Autodesk Fusion 360 part; units mm, degrees
(part 3 of 8)
sketch "Sketch2 (3)" plane through (0, 0, 5) normal (0, 0, 1) x (-1, 0, 0)
  arc A0 (-62.44, 3.6948) -> (-62.5051, 2.3488) centre (0, 0) ccw
  spline S0 degree 3 poles (-62.6664, 2.1601) (-62.6409, 2.1651) (-62.6165, 2.1751) (-62.5731, 2.2037) (-62.5543, 2.2222) (-62.5291, 2.2592) (-62.5208, 2.2761) (-62.5091, 2.3116) (-62.5058, 2.3301) (-62.5051, 2.3488) knots 0 0 0 0 0.007813 0.007813 0.015626 0.015626 0.021241 0.021241 0.026855 0.026855 0.026855 0.026855
  spline S1 degree 5 poles (-62.6664, 2.1601) (-62.6671, 2.1599) (-62.685, 2.1564) (-62.72, 2.1495) (-62.7722, 2.139) (-62.8416, 2.1247) (-62.9274, 2.1065) (-63.0131, 2.0878) (-63.0988, 2.0687) (-63.1845, 2.049) (-63.2701, 2.0289) (-63.3557, 2.0082) (-63.4413, 1.9872) (-63.5268, 1.9656) (-63.6123, 1.9436) (-63.6978, 1.9212) (-63.7832, 1.8983) (-63.8686, 1.875) (-63.954, 1.8513) (-64.0393, 1.8272) (-64.1245, 1.8027) (-64.2097, 1.7777) (-64.2949, 1.7524) (-64.3801, 1.7266) (-64.4651, 1.7005) (-64.5502, 1.674) (-64.6352, 1.647) (-64.7202, 1.6198) (-64.8051, 1.5921) (-64.89, 1.5641) (-64.9748, 1.5357) (-65.0596, 1.5069) (-65.1443, 1.4778) (-65.229, 1.4483) (-65.3136, 1.4184) (-65.3982, 1.3882) (-65.4828, 1.3577) (-65.5673, 1.3268) (-65.6517, 1.2955) (-65.7361, 1.264) (-65.8205, 1.2321) (-65.9047, 1.1998) (-65.989, 1.1672) (-66.0732, 1.1343) (-66.1573, 1.1011) (-66.2414, 1.0675) (-66.3255, 1.0336) (-66.4094, 0.9994) (-66.4934, 0.9649) (-66.5772, 0.93) (-66.6611, 0.8949) (-66.7448, 0.8594) (-66.8285, 0.8236) (-66.8955, 0.7947) (-66.9456, 0.7729) (-66.9791, 0.7583) (-66.9958, 0.751) knots 0.270845 0.270845 0.270845 0.270845 0.270845 0.270845 0.271429 0.285714 0.3 0.314286 0.328571 0.342857 0.357143 0.371429 0.385714 0.4 0.414286 0.428571 0.442857 0.457143 0.471429 0.485714 0.5 0.514286 0.528571 0.542857 0.557143 0.571429 0.585714 0.6 0.614286 0.628571 0.642857 0.657143 0.671429 0.685714 0.7 0.714286 0.728571 0.742857 0.757143 0.771429 0.785714 0.8 0.814286 0.828571 0.842857 0.857143 0.871429 0.885714 0.9 0.914286 0.928571 0.942857 0.957143 0.971429 0.985714 1 1 1 1 1 1
  arc A1 (-66.9958, 0.751) -> (-66.9958, -0.751) centre (0, 0) ccw
  spline S2 degree 5 poles (-66.9958, -0.751) (-66.9791, -0.7583) (-66.9456, -0.7729) (-66.8955, -0.7947) (-66.8285, -0.8236) (-66.7448, -0.8594) (-66.6611, -0.8949) (-66.5772, -0.93) (-66.4934, -0.9649) (-66.4094, -0.9994) (-66.3255, -1.0336) (-66.2414, -1.0675) (-66.1573, -1.1011) (-66.0732, -1.1343) (-65.989, -1.1672) (-65.9047, -1.1998) (-65.8205, -1.2321) (-65.7361, -1.264) (-65.6517, -1.2955) (-65.5673, -1.3268) (-65.4828, -1.3577) (-65.3982, -1.3882) (-65.3136, -1.4184) (-65.229, -1.4483) (-65.1443, -1.4778) (-65.0596, -1.5069) (-64.9748, -1.5357) (-64.89, -1.5641) (-64.8051, -1.5921) (-64.7202, -1.6198) (-64.6352, -1.647) (-64.5502, -1.674) (-64.4651, -1.7005) (-64.3801, -1.7266) (-64.2949, -1.7524) (-64.2097, -1.7777) (-64.1245, -1.8027) (-64.0393, -1.8272) (-63.954, -1.8513) (-63.8686, -1.875) (-63.7832, -1.8983) (-63.6978, -1.9212) (-63.6123, -1.9436) (-63.5268, -1.9656) (-63.4413, -1.9872) (-63.3557, -2.0082) (-63.2701, -2.0289) (-63.1845, -2.049) (-63.0988, -2.0687) (-63.0131, -2.0878) (-62.9274, -2.1065) (-62.8416, -2.1247) (-62.7722, -2.139) (-62.72, -2.1495) (-62.685, -2.1564) (-62.6671, -2.1599) (-62.6664, -2.1601) knots -1 -1 -1 -1 -1 -1 -0.985714 -0.971429 -0.957143 -0.942857 -0.928571 -0.914286 -0.9 -0.885714 -0.871429 -0.857143 -0.842857 -0.828571 -0.814286 -0.8 -0.785714 -0.771429 -0.757143 -0.742857 -0.728571 -0.714286 -0.7 -0.685714 -0.671429 -0.657143 -0.642857 -0.628571 -0.614286 -0.6 -0.585714 -0.571429 -0.557143 -0.542857 -0.528571 -0.514286 -0.5 -0.485714 -0.471429 -0.457143 -0.442857 -0.428571 -0.414286 -0.4 -0.385714 -0.371429 -0.357143 -0.342857 -0.328571 -0.314286 -0.3 -0.285714 -0.271429 -0.270845 -0.270845 -0.270845 -0.270845 -0.270845 -0.270845
  spline S3 degree 3 poles (-62.5051, -2.3488) (-62.5061, -2.3228) (-62.5121, -2.2972) (-62.5337, -2.2498) (-62.549, -2.2284) (-62.5816, -2.1978) (-62.597, -2.1869) (-62.6303, -2.1698) (-62.6481, -2.1637) (-62.6664, -2.1601) knots 0 0 0 0 0.007813 0.007813 0.015626 0.015626 0.021241 0.021241 0.026855 0.026855 0.026855 0.026855
  arc A2 (-62.5051, -2.3488) -> (-62.44, -3.6948) centre (0, 0) ccw
  spline S4 degree 3 poles (-62.5823, -3.8982) (-62.5574, -3.8907) (-62.5341, -3.8785) (-62.4936, -3.8457) (-62.4768, -3.8255) (-62.4553, -3.7863) (-62.4486, -3.7687) (-62.4404, -3.7322) (-62.4389, -3.7134) (-62.44, -3.6948) knots 0 0 0 0 0.007813 0.007813 0.015626 0.015626 0.021241 0.021241 0.026855 0.026855 0.026855 0.026855
  spline S5 degree 5 poles (-62.5823, -3.8982) (-62.583, -3.8984) (-62.6005, -3.9036) (-62.6347, -3.9139) (-62.6856, -3.9294) (-62.7533, -3.9503) (-62.8369, -3.9767) (-62.9204, -4.0035) (-63.0039, -4.0309) (-63.0873, -4.0587) (-63.1706, -4.0871) (-63.2538, -4.1158) (-63.3369, -4.1451) (-63.42, -4.1748) (-63.503, -4.2049) (-63.5859, -4.2355) (-63.6687, -4.2665) (-63.7514, -4.2979) (-63.8341, -4.3298) (-63.9166, -4.362) (-63.9991, -4.3947) (-64.0816, -4.4277) (-64.1639, -4.4612) (-64.2461, -4.495) (-64.3283, -4.5292) (-64.4104, -4.5638) (-64.4924, -4.5988) (-64.5744, -4.6342) (-64.6562, -4.6699) (-64.738, -4.706) (-64.8197, -4.7425) (-64.9013, -4.7793) (-64.9828, -4.8165) (-65.0643, -4.854) (-65.1456, -4.8919) (-65.2269, -4.9301) (-65.3081, -4.9687) (-65.3892, -5.0076) (-65.4703, -5.0468) (-65.5512, -5.0864) (-65.6321, -5.1263) (-65.7129, -5.1665) (-65.7936, -5.2071) (-65.8742, -5.248) (-65.9547, -5.2892) (-66.0352, -5.3307) (-66.1156, -5.3725) (-66.1959, -5.4147) (-66.2761, -5.4572) (-66.3562, -5.5) (-66.4362, -5.543) (-66.5162, -5.5864) (-66.5961, -5.6301) (-66.6599, -5.6653) (-66.7077, -5.6919) (-66.7396, -5.7096) (-66.7555, -5.7185) knots 0.270845 0.270845 0.270845 0.270845 0.270845 0.270845 0.271429 0.285714 0.3 0.314286 0.328571 0.342857 0.357143 0.371429 0.385714 0.4 0.414286 0.428571 0.442857 0.457143 0.471429 0.485714 0.5 0.514286 0.528571 0.542857 0.557143 0.571429 0.585714 0.6 0.614286 0.628571 0.642857 0.657143 0.671429 0.685714 0.7 0.714286 0.728571 0.742857 0.757143 0.771429 0.785714 0.8 0.814286 0.828571 0.842857 0.857143 0.871429 0.885714 0.9 0.914286 0.928571 0.942857 0.957143 0.971429 0.985714 1 1 1 1 1 1
  arc A3 (-66.7555, -5.7185) -> (-66.6105, -7.2135) centre (0, 0) ccw
  spline S6 degree 5 poles (-66.6105, -7.2135) (-66.5932, -7.2192) (-66.5585, -7.2305) (-66.5065, -7.2474) (-66.4371, -7.2696) (-66.3503, -7.2972) (-66.2635, -7.3244) (-66.1767, -7.3513) (-66.0898, -7.3779) (-66.003, -7.4042) (-65.9161, -7.4301) (-65.8291, -7.4557) (-65.7422, -7.481) (-65.6553, -7.506) (-65.5683, -7.5306) (-65.4813, -7.5549) (-65.3943, -7.5789) (-65.3072, -7.6025) (-65.2202, -7.6258) (-65.1331, -7.6487) (-65.046, -7.6713) (-64.9589, -7.6936) (-64.8718, -7.7155) (-64.7847, -7.737) (-64.6976, -7.7582) (-64.6104, -7.779) (-64.5233, -7.7995) (-64.4361, -7.8195) (-64.3489, -7.8393) (-64.2617, -7.8586) (-64.1745, -7.8776) (-64.0873, -7.8961) (-64.0001, -7.9143) (-63.9129, -7.9321) (-63.8256, -7.9495) (-63.7384, -7.9666) (-63.6512, -7.9832) (-63.5639, -7.9994) (-63.4767, -8.0151) (-63.3895, -8.0305) (-63.3022, -8.0454) (-63.215, -8.0599) (-63.1278, -8.074) (-63.0406, -8.0877) (-62.9534, -8.1008) (-62.8662, -8.1136) (-62.779, -8.1258) (-62.6918, -8.1376) (-62.6046, -8.1489) (-62.5174, -8.1597) (-62.4303, -8.1701) (-62.3432, -8.1799) (-62.2727, -8.1874) (-62.2198, -8.1928) (-62.1842, -8.1963) (-62.1661, -8.1981) (-62.1654, -8.1982) knots -1 -1 -1 -1 -1 -1 -0.985714 -0.971429 -0.957143 -0.942857 -0.928571 -0.914286 -0.9 -0.885714 -0.871429 -0.857143 -0.842857 -0.828571 -0.814286 -0.8 -0.785714 -0.771429 -0.757143 -0.742857 -0.728571 -0.714286 -0.7 -0.685714 -0.671429 -0.657143 -0.642857 -0.628571 -0.614286 -0.6 -0.585714 -0.571429 -0.557143 -0.542857 -0.528571 -0.514286 -0.5 -0.485714 -0.471429 -0.457143 -0.442857 -0.428571 -0.414286 -0.4 -0.385714 -0.371429 -0.357143 -0.342857 -0.328571 -0.314286 -0.3 -0.285714 -0.271429 -0.270845 -0.270845 -0.270845 -0.270845 -0.270845 -0.270845
  spline S7 degree 3 poles (-61.9866, -8.3705) (-61.9901, -8.3447) (-61.9986, -8.3198) (-62.0246, -8.2747) (-62.0419, -8.2549) (-62.0773, -8.2275) (-62.0937, -8.2182) (-62.1285, -8.2044) (-62.1468, -8.2) (-62.1654, -8.1982) knots 0 0 0 0 0.007813 0.007813 0.015626 0.015626 0.021241 0.021241 0.026855 0.026855 0.026855 0.026855
  arc A4 (-61.9866, -8.3705) -> (-61.7919, -9.7038) centre (0, 0) ccw
  spline S8 degree 3 poles (-61.914, -9.9201) (-61.8898, -9.9102) (-61.8679, -9.8958) (-61.8307, -9.8593) (-61.8159, -9.8376) (-61.7983, -9.7964) (-61.7933, -9.7783) (-61.7887, -9.7411) (-61.789, -9.7223) (-61.7919, -9.7038) knots 0 0 0 0 0.007813 0.007813 0.015626 0.015626 0.021241 0.021241 0.026855 0.026855 0.026855 0.026855
  spline S9 degree 5 poles (-61.914, -9.9201) (-61.9146, -9.9203) (-61.9315, -9.9272) (-61.9645, -9.9407) (-62.0137, -9.9611) (-62.0791, -9.9884) (-62.1597, -10.0227) (-62.2403, -10.0576) (-62.3207, -10.0928) (-62.401, -10.1286) (-62.4812, -10.1648) (-62.5613, -10.2015) (-62.6412, -10.2386) (-62.721, -10.2762) (-62.8007, -10.3142) (-62.8802, -10.3526) (-62.9597, -10.3915) (-63.039, -10.4308) (-63.1182, -10.4704) (-63.1973, -10.5105) (-63.2762, -10.551) (-63.3551, -10.5918) (-63.4338, -10.633) (-63.5124, -10.6747) (-63.5909, -10.7167) (-63.6693, -10.759) (-63.7475, -10.8018) (-63.8256, -10.8449) (-63.9037, -10.8884) (-63.9816, -10.9322) (-64.0594, -10.9763) (-64.137, -11.0209) (-64.2146, -11.0657) (-64.292, -11.111) (-64.3694, -11.1565) (-64.4466, -11.2024) (-64.5237, -11.2486) (-64.6007, -11.2952) (-64.6775, -11.342) (-64.7543, -11.3892) (-64.8309, -11.4368) (-64.9075, -11.4846) (-64.9839, -11.5328) (-65.0602, -11.5813) (-65.1364, -11.63) (-65.2124, -11.6791) (-65.2884, -11.7285) (-65.3642, -11.7783) (-65.44, -11.8283) (-65.5156, -11.8786) (-65.5911, -11.9292) (-65.6665, -11.9801) (-65.7418, -12.0313) (-65.8019, -12.0725) (-65.847, -12.1035) (-65.877, -12.1243) (-65.892, -12.1347) knots 0.270845 0.270845 0.270845 0.270845 0.270845 0.270845 0.271429 0.285714 0.3 0.314286 0.328571 0.342857 0.357143 0.371429 0.385714 0.4 0.414286 0.428571 0.442857 0.457143 0.471429 0.485714 0.5 0.514286 0.528571 0.542857 0.557143 0.571429 0.585714 0.6 0.614286 0.628571 0.642857 0.657143 0.671429 0.685714 0.7 0.714286 0.728571 0.742857 0.757143 0.771429 0.785714 0.8 0.814286 0.828571 0.842857 0.857143 0.871429 0.885714 0.9 0.914286 0.928571 0.942857 0.957143 0.971429 0.985714 1 1 1 1 1 1
  arc A5 (-65.892, -12.1347) -> (-65.6034, -13.6087) centre (0, 0) ccw
  spline S10 degree 5 poles (-65.6034, -13.6087) (-65.5856, -13.6127) (-65.55, -13.6206) (-65.4965, -13.6323) (-65.4253, -13.6478) (-65.3363, -13.6668) (-65.2473, -13.6856) (-65.1582, -13.704) (-65.0692, -13.722) (-64.9802, -13.7398) (-64.8912, -13.7572) (-64.8023, -13.7744) (-64.7133, -13.7911) (-64.6243, -13.8076) (-64.5354, -13.8237) (-64.4464, -13.8395) (-64.3575, -13.855) (-64.2686, -13.8701) (-64.1797, -13.8849) (-64.0908, -13.8993) (-64.002, -13.9134) (-63.9132, -13.9271) (-63.8243, -13.9405) (-63.7355, -13.9535) (-63.6468, -13.9662) (-63.558, -13.9785) (-63.4693, -13.9904) (-63.3806, -14.002) (-63.2919, -14.0132) (-63.2032, -14.0241) (-63.1146, -14.0345) (-63.026, -14.0446) (-62.9375, -14.0543) (-62.8489, -14.0636) (-62.7604, -14.0725) (-62.672, -14.081) (-62.5835, -14.0891) (-62.4952, -14.0968) (-62.4068, -14.1041) (-62.3185, -14.111) (-62.2302, -14.1174) (-62.142, -14.1235) (-62.0538, -14.129) (-61.9657, -14.1342) (-61.8776, -14.1389) (-61.7896, -14.1432) (-61.7016, -14.1469) (-61.6137, -14.1503) (-61.5258, -14.1531) (-61.438, -14.1554) (-61.3503, -14.1573) (-61.2626, -14.1587) (-61.1918, -14.1594) (-61.1386, -14.1596) (-61.1029, -14.1597) (-61.0847, -14.1597) (-61.0839, -14.1597) knots -1 -1 -1 -1 -1 -1 -0.985714 -0.971429 -0.957143 -0.942857 -0.928571 -0.914286 -0.9 -0.885714 -0.871429 -0.857143 -0.842857 -0.828571 -0.814286 -0.8 -0.785714 -0.771429 -0.757143 -0.742857 -0.728571 -0.714286 -0.7 -0.685714 -0.671429 -0.657143 -0.642857 -0.628571 -0.614286 -0.6 -0.585714 -0.571429 -0.557143 -0.542857 -0.528571 -0.514286 -0.5 -0.485714 -0.471429 -0.457143 -0.442857 -0.428571 -0.414286 -0.4 -0.385714 -0.371429 -0.357143 -0.342857 -0.328571 -0.314286 -0.3 -0.285714 -0.271429 -0.270845 -0.270845 -0.270845 -0.270845 -0.270845 -0.270845
  spline S11 degree 3 poles (-60.8894, -14.314) (-60.8953, -14.2886) (-60.9062, -14.2647) (-60.9364, -14.2223) (-60.9556, -14.2042) (-60.9935, -14.1804) (-61.0106, -14.1727) (-61.0466, -14.1624) (-61.0652, -14.1597) (-61.0839, -14.1597) knots 0 0 0 0 0.007813 0.007813 0.015626 0.015626 0.021241 0.021241 0.026855 0.026855 0.026855 0.026855
  arc A6 (-60.8894, -14.314) -> (-60.5669, -15.6223) centre (0, 0) ccw
  spline S12 degree 3 poles (-60.6675, -15.8493) (-60.6444, -15.8372) (-60.624, -15.8207) (-60.5905, -15.7808) (-60.5778, -15.7577) (-60.5643, -15.7151) (-60.5611, -15.6965) (-60.5601, -15.6591) (-60.5622, -15.6404) (-60.5669, -15.6223) knots 0 0 0 0 0.007813 0.007813 0.015626 0.015626 0.021241 0.021241 0.026855 0.026855 0.026855 0.026855
  spline S13 degree 5 poles (-60.6675, -15.8493) (-60.6681, -15.8496) (-60.6843, -15.8581) (-60.7158, -15.8748) (-60.7629, -15.8998) (-60.8252, -15.9333) (-60.9022, -15.9752) (-60.9791, -16.0177) (-61.0557, -16.0605) (-61.1322, -16.1039) (-61.2085, -16.1477) (-61.2846, -16.1919) (-61.3606, -16.2366) (-61.4364, -16.2817) (-61.512, -16.3272) (-61.5875, -16.3731) (-61.6628, -16.4195) (-61.738, -16.4662) (-61.813, -16.5133) (-61.8878, -16.5608) (-61.9625, -16.6087) (-62.037, -16.657) (-62.1114, -16.7057) (-62.1856, -16.7547) (-62.2597, -16.804) (-62.3336, -16.8538) (-62.4074, -16.9039) (-62.481, -16.9543) (-62.5545, -17.0051) (-62.6278, -17.0563) (-62.7009, -17.1077) (-62.7739, -17.1595) (-62.8468, -17.2117) (-62.9195, -17.2642) (-62.9921, -17.317) (-63.0645, -17.3701) (-63.1368, -17.4235) (-63.2089, -17.4773) (-63.2809, -17.5314) (-63.3528, -17.5858) (-63.4245, -17.6405) (-63.496, -17.6955) (-63.5674, -17.7508) (-63.6387, -17.8064) (-63.7098, -17.8623) (-63.7808, -17.9185) (-63.8516, -17.975) (-63.9223, -18.0318) (-63.9929, -18.0889) (-64.0633, -18.1463) (-64.1336, -18.204) (-64.2037, -18.2619) (-64.2737, -18.3201) (-64.3296, -18.3669) (-64.3714, -18.4022) (-64.3993, -18.4257) (-64.4132, -18.4375) knots 0.270845 0.270845 0.270845 0.270845 0.270845 0.270845 0.271429 0.285714 0.3 0.314286 0.328571 0.342857 0.357143 0.371429 0.385714 0.4 0.414286 0.428571 0.442857 0.457143 0.471429 0.485714 0.5 0.514286 0.528571 0.542857 0.557143 0.571429 0.585714 0.6 0.614286 0.628571 0.642857 0.657143 0.671429 0.685714 0.7 0.714286 0.728571 0.742857 0.757143 0.771429 0.785714 0.8 0.814286 0.828571 0.842857 0.857143 0.871429 0.885714 0.9 0.914286 0.928571 0.942857 0.957143 0.971429 0.985714 1 1 1 1 1 1
  arc A7 (-64.4132, -18.4375) -> (-63.9837, -19.8768) centre (0, 0) ccw
  spline S14 degree 5 poles (-63.9837, -19.8768) (-63.9656, -19.879) (-63.9294, -19.8835) (-63.8751, -19.89) (-63.8027, -19.8985) (-63.7122, -19.9089) (-63.6218, -19.9189) (-63.5314, -19.9287) (-63.4411, -19.9381) (-63.3508, -19.9472) (-63.2605, -19.9559) (-63.1703, -19.9644) (-63.0801, -19.9725) (-62.99, -19.9803) (-62.8999, -19.9877) (-62.8099, -19.9949) (-62.7199, -20.0017) (-62.6299, -20.0081) (-62.54, -20.0143) (-62.4502, -20.0201) (-62.3604, -20.0255) (-62.2706, -20.0306) (-62.1809, -20.0353) (-62.0913, -20.0397) (-62.0017, -20.0438) (-61.9122, -20.0475) (-61.8227, -20.0508) (-61.7333, -20.0538) (-61.644, -20.0564) (-61.5547, -20.0586) (-61.4655, -20.0604) (-61.3763, -20.0619) (-61.2872, -20.063) (-61.1982, -20.0637) (-61.1093, -20.0641) (-61.0204, -20.064) (-60.9316, -20.0635) (-60.8429, -20.0627) (-60.7542, -20.0614) (-60.6657, -20.0597) (-60.5772, -20.0576) (-60.4888, -20.0551) (-60.4005, -20.0521) (-60.3123, -20.0488) (-60.2242, -20.045) (-60.1361, -20.0407) (-60.0482, -20.036) (-59.9604, -20.0308) (-59.8726, -20.0251) (-59.785, -20.019) (-59.6975, -20.0124) (-59.6101, -20.0053) (-59.5396, -19.9991) (-59.4866, -19.9943) (-59.451, -19.9909) (-59.4329, -19.9891) (-59.4322, -19.9891) knots -1 -1 -1 -1 -1 -1 -0.985714 -0.971429 -0.957143 -0.942857 -0.928571 -0.914286 -0.9 -0.885714 -0.871429 -0.857143 -0.842857 -0.828571 -0.814286 -0.8 -0.785714 -0.771429 -0.757143 -0.742857 -0.728571 -0.714286 -0.7 -0.685714 -0.671429 -0.657143 -0.642857 -0.628571 -0.614286 -0.6 -0.585714 -0.571429 -0.557143 -0.542857 -0.528571 -0.514286 -0.5 -0.485714 -0.471429 -0.457143 -0.442857 -0.428571 -0.414286 -0.4 -0.385714 -0.371429 -0.357143 -0.342857 -0.328571 -0.314286 -0.3 -0.285714 -0.271429 -0.270845 -0.270845 -0.270845 -0.270845 -0.270845 -0.270845
  spline S15 degree 3 poles (-59.2236, -20.1238) (-59.232, -20.0991) (-59.2451, -20.0764) (-59.2793, -20.0371) (-59.3001, -20.021) (-59.3401, -20.001) (-59.3579, -19.995) (-59.3947, -19.9881) (-59.4135, -19.9873) (-59.4322, -19.9891) knots 0 0 0 0 0.007813 0.007813 0.015626 0.015626 0.021241 0.021241 0.026855 0.026855 0.026855 0.026855
  arc A8 (-59.2236, -20.1238) -> (-58.7764, -21.3949) centre (0, 0) ccw
  spline S16 degree 3 poles (-58.8546, -21.6306) (-58.8328, -21.6163) (-58.814, -21.5979) (-58.7846, -21.5549) (-58.7742, -21.5308) (-58.7648, -21.487) (-58.7635, -21.4683) (-58.766, -21.4309) (-58.77, -21.4125) (-58.7764, -21.3949) knots 0 0 0 0 0.007813 0.007813 0.015626 0.015626 0.021241 0.021241 0.026855 0.026855 0.026855 0.026855
  spline S17 degree 5 poles (-58.8546, -21.6306) (-58.8552, -21.631) (-58.8704, -21.641) (-58.9003, -21.6606) (-58.9447, -21.69) (-59.0035, -21.7294) (-59.0761, -21.7786) (-59.1485, -21.8282) (-59.2206, -21.8783) (-59.2925, -21.9288) (-59.3643, -21.9798) (-59.4358, -22.0311) (-59.5071, -22.0829) (-59.5782, -22.1351) (-59.6491, -22.1878) (-59.7198, -22.2408) (-59.7903, -22.2941) (-59.8606, -22.3479) (-59.9307, -22.402) (-60.0006, -22.4566) (-60.0703, -22.5114) (-60.1398, -22.5667) (-60.2091, -22.6223) (-60.2783, -22.6782) (-60.3472, -22.7345) (-60.416, -22.7912) (-60.4846, -22.8481) (-60.553, -22.9055) (-60.6212, -22.9631) (-60.6892, -23.0211) (-60.7571, -23.0794) (-60.8248, -23.138) (-60.8923, -23.1969) (-60.9596, -23.2562) (-61.0267, -23.3157) (-61.0937, -23.3756) (-61.1605, -23.4358) (-61.2271, -23.4962) (-61.2935, -23.557) (-61.3597, -23.6181) (-61.4258, -23.6795) (-61.4917, -23.7411) (-61.5575, -23.8031) (-61.623, -23.8653) (-61.6884, -23.9278) (-61.7537, -23.9906) (-61.8187, -24.0537) (-61.8836, -24.117) (-61.9483, -24.1807) (-62.0129, -24.2446) (-62.0772, -24.3088) (-62.1414, -24.3732) (-62.2055, -24.4379) (-62.2566, -24.4899) (-62.2948, -24.529) (-62.3203, -24.5551) (-62.333, -24.5682) knots 0.270845 0.270845 0.270845 0.270845 0.270845 0.270845 0.271429 0.285714 0.3 0.314286 0.328571 0.342857 0.357143 0.371429 0.385714 0.4 0.414286 0.428571 0.442857 0.457143 0.471429 0.485714 0.5 0.514286 0.528571 0.542857 0.557143 0.571429 0.585714 0.6 0.614286 0.628571 0.642857 0.657143 0.671429 0.685714 0.7 0.714286 0.728571 0.742857 0.757143 0.771429 0.785714 0.8 0.814286 0.828571 0.842857 0.857143 0.871429 0.885714 0.9 0.914286 0.928571 0.942857 0.957143 0.971429 0.985714 1 1 1 1 1 1
  arc A9 (-62.333, -24.5682) -> (-61.7666, -25.9593) centre (0, 0) ccw
  spline S18 degree 5 poles (-61.7666, -25.9593) (-61.7484, -25.9598) (-61.7119, -25.9607) (-61.6572, -25.962) (-61.5843, -25.9635) (-61.4933, -25.9651) (-61.4023, -25.9663) (-61.3114, -25.9673) (-61.2206, -25.9679) (-61.1299, -25.9683) (-61.0392, -25.9683) (-60.9486, -25.968) (-60.858, -25.9674) (-60.7676, -25.9664) (-60.6772, -25.9652) (-60.5869, -25.9636) (-60.4966, -25.9616) (-60.4065, -25.9594) (-60.3164, -25.9568) (-60.2264, -25.9539) (-60.1365, -25.9507) (-60.0467, -25.9471) (-59.957, -25.9431) (-59.8673, -25.9389) (-59.7778, -25.9342) (-59.6883, -25.9293) (-59.5989, -25.9239) (-59.5096, -25.9183) (-59.4205, -25.9122) (-59.3314, -25.9058) (-59.2424, -25.8991) (-59.1535, -25.8919) (-59.0647, -25.8844) (-58.9761, -25.8765) (-58.8875, -25.8683) (-58.7991, -25.8596) (-58.7107, -25.8506) (-58.6225, -25.8412) (-58.5344, -25.8314) (-58.4464, -25.8211) (-58.3586, -25.8105) (-58.2708, -25.7995) (-58.1832, -25.788) (-58.0957, -25.7761) (-58.0084, -25.7638) (-57.9212, -25.7511) (-57.8341, -25.7379) (-57.7472, -25.7243) (-57.6604, -25.7102) (-57.5738, -25.6956) (-57.4874, -25.6806) (-57.4011, -25.6651) (-57.3315, -25.6522) (-57.2791, -25.6422) (-57.2441, -25.6354) (-57.2262, -25.6319) (-57.2255, -25.6318) knots -1 -1 -1 -1 -1 -1 -0.985714 -0.971429 -0.957143 -0.942857 -0.928571 -0.914286 -0.9 -0.885714 -0.871429 -0.857143 -0.842857 -0.828571 -0.814286 -0.8 -0.785714 -0.771429 -0.757143 -0.742857 -0.728571 -0.714286 -0.7 -0.685714 -0.671429 -0.657143 -0.642857 -0.628571 -0.614286 -0.6 -0.585714 -0.571429 -0.557143 -0.542857 -0.528571 -0.514286 -0.5 -0.485714 -0.471429 -0.457143 -0.442857 -0.428571 -0.414286 -0.4 -0.385714 -0.371429 -0.357143 -0.342857 -0.328571 -0.314286 -0.3 -0.285714 -0.271429 -0.270845 -0.270845 -0.270845 -0.270845 -0.270845 -0.270845
  spline S19 degree 3 poles (-57.0049, -25.7458) (-57.0156, -25.722) (-57.0309, -25.7006) (-57.0687, -25.6648) (-57.091, -25.6508) (-57.1327, -25.6347) (-57.1511, -25.6305) (-57.1883, -25.6272) (-57.2071, -25.6282) (-57.2255, -25.6318) knots 0 0 0 0 0.007813 0.007813 0.015626 0.015626 0.021241 0.021241 0.026855 0.026855 0.026855 0.026855
  arc A10 (-57.0049, -25.7458) -> (-56.4371, -26.9678) centre (0, 0) ccw
  spline S20 degree 3 poles (-56.4922, -27.2099) (-56.4719, -27.1936) (-56.455, -27.1734) (-56.4298, -27.1278) (-56.4218, -27.1028) (-56.4167, -27.0583) (-56.4172, -27.0395) (-56.4233, -27.0026) (-56.429, -26.9847) (-56.4371, -26.9678) knots 0 0 0 0 0.007813 0.007813 0.015626 0.015626 0.021241 0.021241 0.026855 0.026855 0.026855 0.026855
  spline S21 degree 5 poles (-56.4922, -27.2099) (-56.4928, -27.2103) (-56.5069, -27.2217) (-56.5347, -27.2442) (-56.5761, -27.2777) (-56.6309, -27.3226) (-56.6984, -27.3786) (-56.7656, -27.435) (-56.8326, -27.4918) (-56.8993, -27.549) (-56.9658, -27.6066) (-57.032, -27.6647) (-57.098, -27.7231) (-57.1637, -27.7819) (-57.2292, -27.8411) (-57.2944, -27.9007) (-57.3594, -27.9607) (-57.4242, -28.021) (-57.4888, -28.0816) (-57.5531, -28.1426) (-57.6172, -28.204) (-57.681, -28.2657) (-57.7447, -28.3277) (-57.8081, -28.3901) (-57.8713, -28.4527) (-57.9343, -28.5158) (-57.9971, -28.5791) (-58.0596, -28.6427) (-58.1219, -28.7067) (-58.1841, -28.771) (-58.246, -28.8355) (-58.3077, -28.9004) (-58.3692, -28.9656) (-58.4304, -29.0311) (-58.4915, -29.0968) (-58.5524, -29.1629) (-58.6131, -29.2292) (-58.6735, -29.2958) (-58.7338, -29.3627) (-58.7938, -29.4299) (-58.8537, -29.4974) (-58.9133, -29.5651) (-58.9728, -29.6331) (-59.032, -29.7014) (-59.0911, -29.7699) (-59.15, -29.8387) (-59.2086, -29.9078) (-59.2671, -29.9771) (-59.3253, -30.0467) (-59.3834, -30.1165) (-59.4413, -30.1866) (-59.499, -30.2569) (-59.5565, -30.3275) (-59.6023, -30.3842) (-59.6366, -30.4268) (-59.6594, -30.4553) (-59.6708, -30.4695) knots 0.270845 0.270845 0.270845 0.270845 0.270845 0.270845 0.271429 0.285714 0.3 0.314286 0.328571 0.342857 0.357143 0.371429 0.385714 0.4 0.414286 0.428571 0.442857 0.457143 0.471429 0.485714 0.5 0.514286 0.528571 0.542857 0.557143 0.571429 0.585714 0.6 0.614286 0.628571 0.642857 0.657143 0.671429 0.685714 0.7 0.714286 0.728571 0.742857 0.757143 0.771429 0.785714 0.8 0.814286 0.828571 0.842857 0.857143 0.871429 0.885714 0.9 0.914286 0.928571 0.942857 0.957143 0.971429 0.985714 1 1 1 1 1 1
  arc A11 (-59.6708, -30.4695) -> (-58.9728, -31.7995) centre (0, 0) ccw
  spline S22 degree 5 poles (-58.9728, -31.7995) (-58.9546, -31.7982) (-58.9182, -31.7956) (-58.8637, -31.7916) (-58.791, -31.786) (-58.7002, -31.7788) (-58.6096, -31.7713) (-58.519, -31.7635) (-58.4286, -31.7554) (-58.3382, -31.7469) (-58.2479, -31.7382) (-58.1578, -31.7291) (-58.0677, -31.7198) (-57.9778, -31.7101) (-57.8879, -31.7001) (-57.7982, -31.6898) (-57.7086, -31.6792) (-57.619, -31.6683) (-57.5296, -31.657) (-57.4403, -31.6454) (-57.3512, -31.6335) (-57.2621, -31.6213) (-57.1732, -31.6087) (-57.0844, -31.5958) (-56.9957, -31.5826) (-56.9071, -31.569) (-56.8187, -31.555) (-56.7304, -31.5408) (-56.6422, -31.5262) (-56.5541, -31.5112) (-56.4662, -31.4959) (-56.3784, -31.4802) (-56.2908, -31.4642) (-56.2033, -31.4478) (-56.116, -31.431) (-56.0288, -31.4138) (-55.9417, -31.3963) (-55.8548, -31.3784) (-55.7681, -31.3602) (-55.6815, -31.3415) (-55.595, -31.3224) (-55.5088, -31.303) (-55.4227, -31.2831) (-55.3368, -31.2629) (-55.251, -31.2422) (-55.1654, -31.2211) (-55.0801, -31.1996) (-54.9949, -31.1776) (-54.9099, -31.1552) (-54.8251, -31.1323) (-54.7405, -31.109) (-54.6561, -31.0853) (-54.588, -31.0657) (-54.5369, -31.0507) (-54.5027, -31.0406) (-54.4852, -31.0354) (-54.4845, -31.0352) knots -1 -1 -1 -1 -1 -1 -0.985714 -0.971429 -0.957143 -0.942857 -0.928571 -0.914286 -0.9 -0.885714 -0.871429 -0.857143 -0.842857 -0.828571 -0.814286 -0.8 -0.785714 -0.771429 -0.757143 -0.742857 -0.728571 -0.714286 -0.7 -0.685714 -0.671429 -0.657143 -0.642857 -0.628571 -0.614286 -0.6 -0.585714 -0.571429 -0.557143 -0.542857 -0.528571 -0.514286 -0.5 -0.485714 -0.471429 -0.457143 -0.442857 -0.428571 -0.414286 -0.4 -0.385714 -0.371429 -0.357143 -0.342857 -0.328571 -0.314286 -0.3 -0.285714 -0.271429 -0.270845 -0.270845 -0.270845 -0.270845 -0.270845 -0.270845
  spline S23 degree 3 poles (-54.254, -31.1273) (-54.2669, -31.1047) (-54.2842, -31.0849) (-54.3253, -31.053) (-54.3488, -31.0411) (-54.3919, -31.0292) (-54.4106, -31.0267) (-54.448, -31.027) (-54.4666, -31.0298) (-54.4845, -31.0352) knots 0 0 0 0 0.007813 0.007813 0.015626 0.015626 0.021241 0.021241 0.026855 0.026855 0.026855 0.026855
  arc A12 (-54.254, -31.1273) -> (-53.5708, -32.2888) centre (0, 0) ccw
  spline S24 degree 3 poles (-53.6023, -32.5351) (-53.5837, -32.5169) (-53.5688, -32.4953) (-53.5482, -32.4475) (-53.5426, -32.4218) (-53.5418, -32.377) (-53.5441, -32.3583) (-53.5538, -32.3222) (-53.5612, -32.3049) (-53.5708, -32.2888) knots 0 0 0 0 0.007813 0.007813 0.015626 0.015626 0.021241 0.021241 0.026855 0.026855 0.026855 0.026855
  spline S25 degree 5 poles (-53.6023, -32.5351) (-53.6028, -32.5356) (-53.6159, -32.5484) (-53.6414, -32.5734) (-53.6793, -32.6108) (-53.7295, -32.6607) (-53.7913, -32.7229) (-53.8527, -32.7856) (-53.9139, -32.8486) (-53.9748, -32.912) (-54.0354, -32.9757) (-54.0957, -33.0399) (-54.1558, -33.1044) (-54.2155, -33.1693) (-54.275, -33.2346) (-54.3342, -33.3002) (-54.3931, -33.3661) (-54.4517, -33.4324) (-54.5101, -33.499) (-54.5683, -33.5659) (-54.6261, -33.6332) (-54.6837, -33.7007) (-54.7411, -33.7686) (-54.7982, -33.8368) (-54.8551, -33.9053) (-54.9117, -33.9741) (-54.968, -34.0432) (-55.0241, -34.1126) (-55.08, -34.1823) (-55.1356, -34.2522) (-55.191, -34.3225) (-55.2462, -34.393) (-55.3011, -34.4638) (-55.3558, -34.5349) (-55.4102, -34.6062) (-55.4644, -34.6778) (-55.5184, -34.7497) (-55.5721, -34.8219) (-55.6257, -34.8943) (-55.679, -34.9669) (-55.732, -35.0399) (-55.7849, -35.113) (-55.8375, -35.1864) (-55.8899, -35.2601) (-55.942, -35.334) (-55.994, -35.4082) (-56.0457, -35.4826) (-56.0972, -35.5572) (-56.1485, -35.6321) (-56.1995, -35.7072) (-56.2504, -35.7826) (-56.301, -35.8582) (-56.3514, -35.934) (-56.3916, -35.9948) (-56.4216, -36.0405) (-56.4416, -36.0711) (-56.4515, -36.0863) knots 0.270845 0.270845 0.270845 0.270845 0.270845 0.270845 0.271429 0.285714 0.3 0.314286 0.328571 0.342857 0.357143 0.371429 0.385714 0.4 0.414286 0.428571 0.442857 0.457143 0.471429 0.485714 0.5 0.514286 0.528571 0.542857 0.557143 0.571429 0.585714 0.6 0.614286 0.628571 0.642857 0.657143 0.671429 0.685714 0.7 0.714286 0.728571 0.742857 0.757143 0.771429 0.785714 0.8 0.814286 0.828571 0.842857 0.857143 0.871429 0.885714 0.9 0.914286 0.928571 0.942857 0.957143 0.971429 0.985714 1 1 1 1 1 1
  arc A13 (-56.4515, -36.0863) -> (-55.6284, -37.3427) centre (0, 0) ccw
  spline S26 degree 5 poles (-55.6284, -37.3427) (-55.6104, -37.3397) (-55.5745, -37.3336) (-55.5205, -37.3243) (-55.4487, -37.3118) (-55.3591, -37.2958) (-55.2696, -37.2796) (-55.1802, -37.2631) (-55.091, -37.2463) (-55.0018, -37.2292) (-54.9128, -37.2118) (-54.824, -37.1941) (-54.7352, -37.176) (-54.6466, -37.1577) (-54.5582, -37.1391) (-54.4698, -37.1202) (-54.3817, -37.101) (-54.2936, -37.0815) (-54.2057, -37.0616) (-54.118, -37.0415) (-54.0304, -37.021) (-53.9429, -37.0002) (-53.8556, -36.9791) (-53.7684, -36.9577) (-53.6814, -36.936) (-53.5946, -36.9139) (-53.5079, -36.8915) (-53.4214, -36.8688) (-53.335, -36.8457) (-53.2488, -36.8223) (-53.1628, -36.7986) (-53.077, -36.7745) (-52.9913, -36.7501) (-52.9058, -36.7253) (-52.8205, -36.7002) (-52.7353, -36.6747) (-52.6504, -36.6489) (-52.5656, -36.6227) (-52.481, -36.5962) (-52.3966, -36.5692) (-52.3125, -36.5419) (-52.2285, -36.5142) (-52.1447, -36.4861) (-52.0611, -36.4577) (-51.9778, -36.4288) (-51.8946, -36.3996) (-51.8117, -36.3699) (-51.7291, -36.3398) (-51.6466, -36.3093) (-51.5644, -36.2784) (-51.4825, -36.247) (-51.4007, -36.2152) (-51.3349, -36.1892) (-51.2855, -36.1693) (-51.2524, -36.1559) (-51.2355, -36.1491) (-51.2348, -36.1488) knots -1 -1 -1 -1 -1 -1 -0.985714 -0.971429 -0.957143 -0.942857 -0.928571 -0.914286 -0.9 -0.885714 -0.871429 -0.857143 -0.842857 -0.828571 -0.814286 -0.8 -0.785714 -0.771429 -0.757143 -0.742857 -0.728571 -0.714286 -0.7 -0.685714 -0.671429 -0.657143 -0.642857 -0.628571 -0.614286 -0.6 -0.585714 -0.571429 -0.557143 -0.542857 -0.528571 -0.514286 -0.5 -0.485714 -0.471429 -0.457143 -0.442857 -0.428571 -0.414286 -0.4 -0.385714 -0.371429 -0.357143 -0.342857 -0.328571 -0.314286 -0.3 -0.285714 -0.271429 -0.270845 -0.270845 -0.270845 -0.270845 -0.270845 -0.270845
  spline S27 degree 3 poles (-50.9965, -36.2183) (-51.0115, -36.1971) (-51.0306, -36.179) (-51.0746, -36.1511) (-51.0992, -36.1416) (-51.1432, -36.1339) (-51.162, -36.1332) (-51.1993, -36.1372) (-51.2175, -36.1418) (-51.2348, -36.1488) knots 0 0 0 0 0.007813 0.007813 0.015626 0.015626 0.021241 0.021241 0.026855 0.026855 0.026855 0.026855
  arc A14 (-50.9965, -36.2183) -> (-50.2044, -37.3084) centre (0, 0) ccw
  spline S28 degree 3 poles (-50.212, -37.5566) (-50.1952, -37.5367) (-50.1825, -37.5137) (-50.1666, -37.4641) (-50.1635, -37.438) (-50.167, -37.3934) (-50.1711, -37.375) (-50.1842, -37.34) (-50.1932, -37.3235) (-50.2044, -37.3084) knots 0 0 0 0 0.007813 0.007813 0.015626 0.015626 0.021241 0.021241 0.026855 0.026855 0.026855 0.026855
  spline S29 degree 5 poles (-50.212, -37.5566) (-50.2125, -37.5572) (-50.2242, -37.5711) (-50.2472, -37.5985) (-50.2813, -37.6393) (-50.3264, -37.6939) (-50.3819, -37.7618) (-50.4371, -37.83) (-50.4919, -37.8987) (-50.5464, -37.9676) (-50.6005, -38.037) (-50.6544, -38.1067) (-50.7079, -38.1767) (-50.7611, -38.247) (-50.814, -38.3177) (-50.8666, -38.3887) (-50.9189, -38.46) (-50.9708, -38.5317) (-51.0225, -38.6036) (-51.0739, -38.6758) (-51.125, -38.7483) (-51.1759, -38.8211) (-51.2264, -38.8942) (-51.2767, -38.9676) (-51.3266, -39.0413) (-51.3763, -39.1152) (-51.4258, -39.1894) (-51.4749, -39.2639) (-51.5238, -39.3387) (-51.5724, -39.4137) (-51.6208, -39.4889) (-51.6689, -39.5645) (-51.7167, -39.6402) (-51.7643, -39.7163) (-51.8116, -39.7925) (-51.8586, -39.869) (-51.9054, -39.9458) (-51.9519, -40.0228) (-51.9982, -40.1) (-52.0442, -40.1775) (-52.09, -40.2552) (-52.1355, -40.3331) (-52.1808, -40.4113) (-52.2259, -40.4897) (-52.2706, -40.5683) (-52.3152, -40.6471) (-52.3595, -40.7261) (-52.4035, -40.8054) (-52.4474, -40.8849) (-52.4909, -40.9646) (-52.5343, -41.0445) (-52.5774, -41.1246) (-52.6202, -41.2049) (-52.6543, -41.2693) (-52.6798, -41.3177) (-52.6967, -41.3501) (-52.7052, -41.3662) knots 0.270845 0.270845 0.270845 0.270845 0.270845 0.270845 0.271429 0.285714 0.3 0.314286 0.328571 0.342857 0.357143 0.371429 0.385714 0.4 0.414286 0.428571 0.442857 0.457143 0.471429 0.485714 0.5 0.514286 0.528571 0.542857 0.557143 0.571429 0.585714 0.6 0.614286 0.628571 0.642857 0.657143 0.671429 0.685714 0.7 0.714286 0.728571 0.742857 0.757143 0.771429 0.785714 0.8 0.814286 0.828571 0.842857 0.857143 0.871429 0.885714 0.9 0.914286 0.928571 0.942857 0.957143 0.971429 0.985714 1 1 1 1 1 1
  arc A15 (-52.7052, -41.3662) -> (-51.7646, -42.5373) centre (0, 0) ccw
  spline S30 degree 5 poles (-51.7646, -42.5373) (-51.747, -42.5326) (-51.7118, -42.523) (-51.659, -42.5086) (-51.5888, -42.4892) (-51.5011, -42.4647) (-51.4136, -42.4399) (-51.3262, -42.4148) (-51.239, -42.3894) (-51.1519, -42.3638) (-51.065, -42.3379) (-50.9783, -42.3117) (-50.8917, -42.2852) (-50.8053, -42.2584) (-50.719, -42.2314) (-50.6329, -42.204) (-50.547, -42.1764) (-50.4613, -42.1485) (-50.3757, -42.1202) (-50.2903, -42.0917) (-50.2051, -42.0629) (-50.12, -42.0338) (-50.0352, -42.0043) (-49.9505, -41.9746) (-49.866, -41.9446) (-49.7817, -41.9142) (-49.6976, -41.8836) (-49.6136, -41.8526) (-49.5299, -41.8213) (-49.4464, -41.7897) (-49.3631, -41.7578) (-49.2799, -41.7255) (-49.197, -41.6929) (-49.1143, -41.66) (-49.0318, -41.6268) (-48.9495, -41.5932) (-48.8674, -41.5593) (-48.7856, -41.5251) (-48.704, -41.4905) (-48.6226, -41.4555) (-48.5414, -41.4202) (-48.4605, -41.3845) (-48.3798, -41.3485) (-48.2994, -41.3121) (-48.2192, -41.2753) (-48.1393, -41.2382) (-48.0597, -41.2007) (-47.9803, -41.1628) (-47.9012, -41.1244) (-47.8223, -41.0857) (-47.7438, -41.0466) (-47.6655, -41.007) (-47.6025, -40.9748) (-47.5552, -40.9503) (-47.5236, -40.9337) (-47.5074, -40.9253) (-47.5068, -40.9249) knots -1 -1 -1 -1 -1 -1 -0.985714 -0.971429 -0.957143 -0.942857 -0.928571 -0.914286 -0.9 -0.885714 -0.871429 -0.857143 -0.842857 -0.828571 -0.814286 -0.8 -0.785714 -0.771429 -0.757143 -0.742857 -0.728571 -0.714286 -0.7 -0.685714 -0.671429 -0.657143 -0.642857 -0.628571 -0.614286 -0.6 -0.585714 -0.571429 -0.557143 -0.542857 -0.528571 -0.514286 -0.5 -0.485714 -0.471429 -0.457143 -0.442857 -0.428571 -0.414286 -0.4 -0.385714 -0.371429 -0.357143 -0.342857 -0.328571 -0.314286 -0.3 -0.285714 -0.271429 -0.270845 -0.270845 -0.270845 -0.270845 -0.270845 -0.270845
  spline S31 degree 3 poles (-47.2628, -40.9711) (-47.2799, -40.9514) (-47.3006, -40.9352) (-47.3471, -40.9118) (-47.3724, -40.9047) (-47.4171, -40.9012) (-47.4358, -40.9024) (-47.4725, -40.9099) (-47.4902, -40.9163) (-47.5068, -40.9249) knots 0 0 0 0 0.007813 0.007813 0.015626 0.015626 0.021241 0.021241 0.026855 0.026855 0.026855 0.026855
  arc A16 (-47.2628, -40.9711) -> (-46.3693, -41.9797) centre (0, 0) ccw
  spline S32 degree 3 poles (-46.3529, -42.2275) (-46.3381, -42.206) (-46.3276, -42.1819) (-46.3166, -42.131) (-46.316, -42.1047) (-46.3238, -42.0606) (-46.3297, -42.0428) (-46.3461, -42.0091) (-46.3567, -41.9936) (-46.3693, -41.9797) knots 0 0 0 0 0.007813 0.007813 0.015626 0.015626 0.021241 0.021241 0.026855 0.026855 0.026855 0.026855
  spline S33 degree 5 poles (-46.3529, -42.2275) (-46.3533, -42.228) (-46.3636, -42.243) (-46.3838, -42.2725) (-46.4138, -42.3165) (-46.4535, -42.3751) (-46.5022, -42.4481) (-46.5505, -42.5213) (-46.5984, -42.5949) (-46.646, -42.6688) (-46.6932, -42.7431) (-46.7401, -42.8176) (-46.7866, -42.8925) (-46.8327, -42.9676) (-46.8786, -43.0431) (-46.9241, -43.1188) (-46.9692, -43.1949) (-47.014, -43.2712) (-47.0586, -43.3478) (-47.1027, -43.4246) (-47.1466, -43.5017) (-47.1902, -43.5791) (-47.2334, -43.6567) (-47.2764, -43.7346) (-47.319, -43.8128) (-47.3613, -43.8912) (-47.4034, -43.9698) (-47.4451, -44.0487) (-47.4866, -44.1278) (-47.5277, -44.2071) (-47.5686, -44.2867) (-47.6091, -44.3665) (-47.6494, -44.4466) (-47.6894, -44.5268) (-47.7291, -44.6073) (-47.7686, -44.688) (-47.8077, -44.7689) (-47.8466, -44.85) (-47.8852, -44.9314) (-47.9236, -45.0129) (-47.9616, -45.0947) (-47.9994, -45.1766) (-48.037, -45.2588) (-48.0742, -45.3412) (-48.1112, -45.4237) (-48.1479, -45.5065) (-48.1844, -45.5894) (-48.2206, -45.6726) (-48.2566, -45.7559) (-48.2922, -45.8394) (-48.3277, -45.9232) (-48.3628, -46.0071) (-48.3977, -46.0911) (-48.4254, -46.1585) (-48.4461, -46.2092) (-48.4599, -46.243) (-48.4667, -46.2599) knots 0.270845 0.270845 0.270845 0.270845 0.270845 0.270845 0.271429 0.285714 0.3 0.314286 0.328571 0.342857 0.357143 0.371429 0.385714 0.4 0.414286 0.428571 0.442857 0.457143 0.471429 0.485714 0.5 0.514286 0.528571 0.542857 0.557143 0.571429 0.585714 0.6 0.614286 0.628571 0.642857 0.657143 0.671429 0.685714 0.7 0.714286 0.728571 0.742857 0.757143 0.771429 0.785714 0.8 0.814286 0.828571 0.842857 0.857143 0.871429 0.885714 0.9 0.914286 0.928571 0.942857 0.957143 0.971429 0.985714 1 1 1 1 1 1
  arc A17 (-48.4667, -46.2599) -> (-47.4175, -47.3347) centre (0, 0) ccw
  spline S34 degree 5 poles (-47.4175, -47.3347) (-47.4005, -47.3283) (-47.3663, -47.3154) (-47.3152, -47.2959) (-47.2471, -47.2699) (-47.1622, -47.237) (-47.0775, -47.2039) (-46.993, -47.1705) (-46.9086, -47.1368) (-46.8244, -47.1029) (-46.7404, -47.0687) (-46.6566, -47.0343) (-46.573, -46.9996) (-46.4896, -46.9646) (-46.4063, -46.9293) (-46.3233, -46.8938) (-46.2404, -46.858) (-46.1578, -46.8219) (-46.0753, -46.7856) (-45.9931, -46.7489) (-45.9111, -46.712) (-45.8292, -46.6748) (-45.7476, -46.6373) (-45.6662, -46.5996) (-45.585, -46.5615) (-45.504, -46.5232) (-45.4232, -46.4845) (-45.3427, -46.4456) (-45.2624, -46.4064) (-45.1823, -46.3669) (-45.1024, -46.3271) (-45.0228, -46.2869) (-44.9434, -46.2465) (-44.8642, -46.2058) (-44.7853, -46.1647) (-44.7067, -46.1234) (-44.6283, -46.0817) (-44.5501, -46.0397) (-44.4722, -45.9974) (-44.3946, -45.9547) (-44.3172, -45.9118) (-44.2401, -45.8684) (-44.1633, -45.8248) (-44.0867, -45.7808) (-44.0105, -45.7365) (-43.9345, -45.6918) (-43.8589, -45.6468) (-43.7835, -45.6014) (-43.7085, -45.5556) (-43.6337, -45.5094) (-43.5593, -45.4629) (-43.4852, -45.416) (-43.4256, -45.3778) (-43.3809, -45.3488) (-43.351, -45.3293) (-43.3358, -45.3193) (-43.3352, -45.319) knots -1 -1 -1 -1 -1 -1 -0.985714 -0.971429 -0.957143 -0.942857 -0.928571 -0.914286 -0.9 -0.885714 -0.871429 -0.857143 -0.842857 -0.828571 -0.814286 -0.8 -0.785714 -0.771429 -0.757143 -0.742857 -0.728571 -0.714286 -0.7 -0.685714 -0.671429 -0.657143 -0.642857 -0.628571 -0.614286 -0.6 -0.585714 -0.571429 -0.557143 -0.542857 -0.528571 -0.514286 -0.5 -0.485714 -0.471429 -0.457143 -0.442857 -0.428571 -0.414286 -0.4 -0.385714 -0.371429 -0.357143 -0.342857 -0.328571 -0.314286 -0.3 -0.285714 -0.271429 -0.270845 -0.270845 -0.270845 -0.270845 -0.270845 -0.270845
  spline S35 degree 3 poles (-43.0879, -45.3413) (-43.1068, -45.3234) (-43.129, -45.3093) (-43.1775, -45.2904) (-43.2034, -45.2858) (-43.2482, -45.2867) (-43.2667, -45.2897) (-43.3025, -45.3007) (-43.3195, -45.3087) (-43.3352, -45.319) knots 0 0 0 0 0.007813 0.007813 0.015626 0.015626 0.021241 0.021241 0.026855 0.026855 0.026855 0.026855
  arc A18 (-43.0879, -45.3413) -> (-42.1012, -46.259) centre (0, 0) ccw
  spline S36 degree 3 poles (-42.0609, -46.504) (-42.0483, -46.4813) (-42.0402, -46.4562) (-42.0341, -46.4045) (-42.0361, -46.3783) (-42.0481, -46.3352) (-42.0557, -46.3179) (-42.0753, -46.2861) (-42.0873, -46.2716) (-42.1012, -46.259) knots 0 0 0 0 0.007813 0.007813 0.015626 0.015626 0.021241 0.021241 0.026855 0.026855 0.026855 0.026855
  spline S37 degree 5 poles (-42.0609, -46.504) (-42.0613, -46.5046) (-42.0701, -46.5206) (-42.0874, -46.5518) (-42.113, -46.5985) (-42.1468, -46.6607) (-42.1883, -46.738) (-42.2293, -46.8156) (-42.2699, -46.8935) (-42.3101, -46.9716) (-42.3499, -47.0501) (-42.3894, -47.1288) (-42.4285, -47.2078) (-42.4671, -47.2871) (-42.5055, -47.3666) (-42.5434, -47.4464) (-42.581, -47.5264) (-42.6183, -47.6067) (-42.6552, -47.6872) (-42.6918, -47.768) (-42.728, -47.8489) (-42.7639, -47.9302) (-42.7994, -48.0116) (-42.8347, -48.0933) (-42.8696, -48.1752) (-42.9041, -48.2573) (-42.9384, -48.3396) (-42.9723, -48.4222) (-43.0059, -48.5049) (-43.0392, -48.5878) (-43.0722, -48.671) (-43.1049, -48.7544) (-43.1373, -48.8379) (-43.1693, -48.9216) (-43.2011, -49.0056) (-43.2326, -49.0897) (-43.2637, -49.174) (-43.2946, -49.2585) (-43.3252, -49.3432) (-43.3555, -49.4281) (-43.3855, -49.5131) (-43.4152, -49.5984) (-43.4446, -49.6838) (-43.4737, -49.7693) (-43.5026, -49.8551) (-43.5312, -49.941) (-43.5595, -50.0271) (-43.5875, -50.1133) (-43.6152, -50.1997) (-43.6426, -50.2863) (-43.6698, -50.3731) (-43.6967, -50.46) (-43.7234, -50.547) (-43.7444, -50.6168) (-43.7601, -50.6692) (-43.7705, -50.7042) (-43.7757, -50.7216) knots 0.270845 0.270845 0.270845 0.270845 0.270845 0.270845 0.271429 0.285714 0.3 0.314286 0.328571 0.342857 0.357143 0.371429 0.385714 0.4 0.414286 0.428571 0.442857 0.457143 0.471429 0.485714 0.5 0.514286 0.528571 0.542857 0.557143 0.571429 0.585714 0.6 0.614286 0.628571 0.642857 0.657143 0.671429 0.685714 0.7 0.714286 0.728571 0.742857 0.757143 0.771429 0.785714 0.8 0.814286 0.828571 0.842857 0.857143 0.871429 0.885714 0.9 0.914286 0.928571 0.942857 0.957143 0.971429 0.985714 1 1 1 1 1 1
  arc A19 (-43.7757, -50.7216) -> (-42.6277, -51.6902) centre (0, 0) ccw
  spline S38 degree 5 poles (-42.6277, -51.6902) (-42.6113, -51.6822) (-42.5786, -51.666) (-42.5296, -51.6417) (-42.4644, -51.6092) (-42.383, -51.5683) (-42.3019, -51.5271) (-42.221, -51.4857) (-42.1403, -51.4441) (-42.0598, -51.4022) (-41.9795, -51.3601) (-41.8994, -51.3177) (-41.8195, -51.2751) (-41.7398, -51.2322) (-41.6604, -51.1891) (-41.5811, -51.1457) (-41.5021, -51.1021) (-41.4233, -51.0582) (-41.3448, -51.0141) (-41.2665, -50.9697) (-41.1884, -50.925) (-41.1105, -50.8801) (-41.0329, -50.8349) (-40.9555, -50.7894) (-40.8783, -50.7437) (-40.8014, -50.6978) (-40.7248, -50.6515) (-40.6484, -50.605) (-40.5722, -50.5582) (-40.4963, -50.5111) (-40.4206, -50.4638) (-40.3453, -50.4162) (-40.2701, -50.3683) (-40.1953, -50.3201) (-40.1207, -50.2716) (-40.0464, -50.2229) (-39.9724, -50.1738) (-39.8987, -50.1245) (-39.8252, -50.0748) (-39.7521, -50.0249) (-39.6792, -49.9746) (-39.6066, -49.9241) (-39.5344, -49.8732) (-39.4624, -49.8221) (-39.3908, -49.7706) (-39.3195, -49.7188) (-39.2486, -49.6667) (-39.1779, -49.6142) (-39.1077, -49.5614) (-39.0377, -49.5082) (-38.9682, -49.4547) (-38.899, -49.4009) (-38.8433, -49.3571) (-38.8016, -49.324) (-38.7737, -49.3017) (-38.7595, -49.2903) (-38.759, -49.2898) knots -1 -1 -1 -1 -1 -1 -0.985714 -0.971429 -0.957143 -0.942857 -0.928571 -0.914286 -0.9 -0.885714 -0.871429 -0.857143 -0.842857 -0.828571 -0.814286 -0.8 -0.785714 -0.771429 -0.757143 -0.742857 -0.728571 -0.714286 -0.7 -0.685714 -0.671429 -0.657143 -0.642857 -0.628571 -0.614286 -0.6 -0.585714 -0.571429 -0.557143 -0.542857 -0.528571 -0.514286 -0.5 -0.485714 -0.471429 -0.457143 -0.442857 -0.428571 -0.414286 -0.4 -0.385714 -0.371429 -0.357143 -0.342857 -0.328571 -0.314286 -0.3 -0.285714 -0.271429 -0.270845 -0.270845 -0.270845 -0.270845 -0.270845 -0.270845
  spline S39 degree 3 poles (-38.5107, -49.2882) (-38.5312, -49.2722) (-38.5547, -49.2603) (-38.6048, -49.2462) (-38.631, -49.2442) (-38.6755, -49.2493) (-38.6937, -49.2541) (-38.7282, -49.2685) (-38.7444, -49.2781) (-38.759, -49.2898) knots 0 0 0 0 0.007813 0.007813 0.015626 0.015626 0.021241 0.021241 0.026855 0.026855 0.026855 0.026855
  arc A20 (-38.5107, -49.2882) -> (-37.44, -50.1064) centre (0, 0) ccw
  spline S40 degree 3 poles (-37.3763, -50.3464) (-37.3659, -50.3225) (-37.3603, -50.2968) (-37.3592, -50.2447) (-37.3637, -50.2189) (-37.3799, -50.1771) (-37.389, -50.1607) (-37.4116, -50.1308) (-37.425, -50.1176) (-37.44, -50.1064) knots 0 0 0 0 0.007813 0.007813 0.015626 0.015626 0.021241 0.021241 0.026855 0.026855 0.026855 0.026855
  spline S41 degree 5 poles (-37.3763, -50.3464) (-37.3766, -50.347) (-37.3838, -50.3637) (-37.398, -50.3965) (-37.419, -50.4455) (-37.4467, -50.5106) (-37.4804, -50.5916) (-37.5138, -50.6727) (-37.5467, -50.7542) (-37.5792, -50.8358) (-37.6113, -50.9178) (-37.6429, -50.9999) (-37.6742, -51.0823) (-37.705, -51.165) (-37.7355, -51.2478) (-37.7656, -51.3309) (-37.7953, -51.4142) (-37.8246, -51.4977) (-37.8536, -51.5814) (-37.8822, -51.6653) (-37.9104, -51.7494) (-37.9383, -51.8337) (-37.9658, -51.9182) (-37.993, -52.0029) (-38.0198, -52.0878) (-38.0463, -52.1729) (-38.0725, -52.2581) (-38.0983, -52.3435) (-38.1238, -52.4291) (-38.1489, -52.5149) (-38.1737, -52.6009) (-38.1982, -52.687) (-38.2223, -52.7733) (-38.2462, -52.8597) (-38.2697, -52.9463) (-38.2929, -53.0331) (-38.3158, -53.12) (-38.3384, -53.2071) (-38.3606, -53.2943) (-38.3826, -53.3817) (-38.4042, -53.4693) (-38.4256, -53.557) (-38.4466, -53.6448) (-38.4674, -53.7328) (-38.4878, -53.8209) (-38.5079, -53.9092) (-38.5278, -53.9976) (-38.5473, -54.0862) (-38.5666, -54.1749) (-38.5856, -54.2637) (-38.6043, -54.3526) (-38.6226, -54.4417) (-38.6407, -54.531) (-38.655, -54.6024) (-38.6656, -54.6561) (-38.6725, -54.6919) (-38.676, -54.7098) knots 0.270845 0.270845 0.270845 0.270845 0.270845 0.270845 0.271429 0.285714 0.3 0.314286 0.328571 0.342857 0.357143 0.371429 0.385714 0.4 0.414286 0.428571 0.442857 0.457143 0.471429 0.485714 0.5 0.514286 0.528571 0.542857 0.557143 0.571429 0.585714 0.6 0.614286 0.628571 0.642857 0.657143 0.671429 0.685714 0.7 0.714286 0.728571 0.742857 0.757143 0.771429 0.785714 0.8 0.814286 0.828571 0.842857 0.857143 0.871429 0.885714 0.9 0.914286 0.928571 0.942857 0.957143 0.971429 0.985714 1 1 1 1 1 1
  arc A21 (-38.676, -54.7098) -> (-37.4399, -55.5631) centre (0, 0) ccw
  spline S42 degree 5 poles (-37.4399, -55.5631) (-37.4244, -55.5535) (-37.3934, -55.5343) (-37.3469, -55.5053) (-37.2851, -55.4667) (-37.2081, -55.4181) (-37.1313, -55.3693) (-37.0548, -55.3203) (-36.9785, -55.2711) (-36.9024, -55.2216) (-36.8265, -55.1719) (-36.7509, -55.122) (-36.6755, -55.0719) (-36.6003, -55.0215) (-36.5254, -54.9709) (-36.4507, -54.9201) (-36.3763, -54.8691) (-36.3021, -54.8178) (-36.2282, -54.7662) (-36.1545, -54.7145) (-36.0811, -54.6625) (-36.0079, -54.6103) (-35.935, -54.5578) (-35.8624, -54.5051) (-35.79, -54.4522) (-35.7179, -54.399) (-35.6461, -54.3456) (-35.5745, -54.2919) (-35.5032, -54.238) (-35.4322, -54.1838) (-35.3615, -54.1294) (-35.2911, -54.0747) (-35.2209, -54.0198) (-35.1511, -53.9646) (-35.0815, -53.9091) (-35.0123, -53.8534) (-34.9433, -53.7975) (-34.8747, -53.7412) (-34.8064, -53.6847) (-34.7384, -53.628) (-34.6707, -53.5709) (-34.6034, -53.5136) (-34.5364, -53.456) (-34.4697, -53.3982) (-34.4034, -53.34) (-34.3374, -53.2816) (-34.2718, -53.2228) (-34.2066, -53.1638) (-34.1417, -53.1044) (-34.0773, -53.0448) (-34.0132, -52.9848) (-33.9495, -52.9246) (-33.8983, -52.8756) (-33.86, -52.8386) (-33.8344, -52.8137) (-33.8214, -52.801) (-33.8209, -52.8005) knots -1 -1 -1 -1 -1 -1 -0.985714 -0.971429 -0.957143 -0.942857 -0.928571 -0.914286 -0.9 -0.885714 -0.871429 -0.857143 -0.842857 -0.828571 -0.814286 -0.8 -0.785714 -0.771429 -0.757143 -0.742857 -0.728571 -0.714286 -0.7 -0.685714 -0.671429 -0.657143 -0.642857 -0.628571 -0.614286 -0.6 -0.585714 -0.571429 -0.557143 -0.542857 -0.528571 -0.514286 -0.5 -0.485714 -0.471429 -0.457143 -0.442857 -0.428571 -0.414286 -0.4 -0.385714 -0.371429 -0.357143 -0.342857 -0.328571 -0.314286 -0.3 -0.285714 -0.271429 -0.270845 -0.270845 -0.270845 -0.270845 -0.270845 -0.270845
  spline S43 degree 3 poles (-33.5739, -52.775) (-33.5959, -52.761) (-33.6204, -52.7514) (-33.6716, -52.7422) (-33.6979, -52.7427) (-33.7417, -52.7521) (-33.7593, -52.7586) (-33.7923, -52.7763) (-33.8075, -52.7874) (-33.8209, -52.8005) knots 0 0 0 0 0.007813 0.007813 0.015626 0.015626 0.021241 0.021241 0.026855 0.026855 0.026855 0.026855
  arc A22 (-33.5739, -52.775) -> (-32.4292, -53.486) centre (0, 0) ccw
  spline S44 degree 3 poles (-32.3427, -53.7187) (-32.3346, -53.6939) (-32.3315, -53.6678) (-32.3355, -53.6159) (-32.3425, -53.5905) (-32.3626, -53.5505) (-32.3733, -53.5351) (-32.3987, -53.5076) (-32.4132, -53.4957) (-32.4292, -53.486) knots 0 0 0 0 0.007813 0.007813 0.015626 0.015626 0.021241 0.021241 0.026855 0.026855 0.026855 0.026855
  spline S45 degree 5 poles (-32.3427, -53.7187) (-32.3429, -53.7194) (-32.3485, -53.7367) (-32.3595, -53.7707) (-32.3757, -53.8214) (-32.3969, -53.889) (-32.4227, -53.9728) (-32.448, -54.0568) (-32.4729, -54.141) (-32.4974, -54.2254) (-32.5214, -54.3101) (-32.545, -54.3949) (-32.5681, -54.48) (-32.5909, -54.5652) (-32.6132, -54.6506) (-32.6351, -54.7362) (-32.6567, -54.8219) (-32.6778, -54.9079) (-32.6986, -54.994) (-32.7189, -55.0803) (-32.7389, -55.1667) (-32.7585, -55.2533) (-32.7778, -55.3401) (-32.7967, -55.427) (-32.8152, -55.5141) (-32.8333, -55.6013) (-32.8511, -55.6887) (-32.8685, -55.7762) (-32.8856, -55.8638) (-32.9024, -55.9516) (-32.9188, -56.0396) (-32.9348, -56.1277) (-32.9506, -56.2159) (-32.9659, -56.3042) (-32.981, -56.3927) (-32.9957, -56.4813) (-33.0101, -56.57) (-33.0242, -56.6589) (-33.0379, -56.7479) (-33.0513, -56.837) (-33.0644, -56.9262) (-33.0772, -57.0156) (-33.0897, -57.105) (-33.1018, -57.1946) (-33.1137, -57.2843) (-33.1252, -57.3741) (-33.1364, -57.464) (-33.1473, -57.554) (-33.1579, -57.6442) (-33.1682, -57.7344) (-33.1782, -57.8248) (-33.188, -57.9152) (-33.1974, -58.0058) (-33.2046, -58.0783) (-33.21, -58.1327) (-33.2135, -58.169) (-33.2152, -58.1872) knots 0.270845 0.270845 0.270845 0.270845 0.270845 0.270845 0.271429 0.285714 0.3 0.314286 0.328571 0.342857 0.357143 0.371429 0.385714 0.4 0.414286 0.428571 0.442857 0.457143 0.471429 0.485714 0.5 0.514286 0.528571 0.542857 0.557143 0.571429 0.585714 0.6 0.614286 0.628571 0.642857 0.657143 0.671429 0.685714 0.7 0.714286 0.728571 0.742857 0.757143 0.771429 0.785714 0.8 0.814286 0.828571 0.842857 0.857143 0.871429 0.885714 0.9 0.914286 0.928571 0.942857 0.957143 0.971429 0.985714 1 1 1 1 1 1
  arc A23 (-33.2152, -58.1872) -> (-31.9025, -58.9172) centre (0, 0) ccw